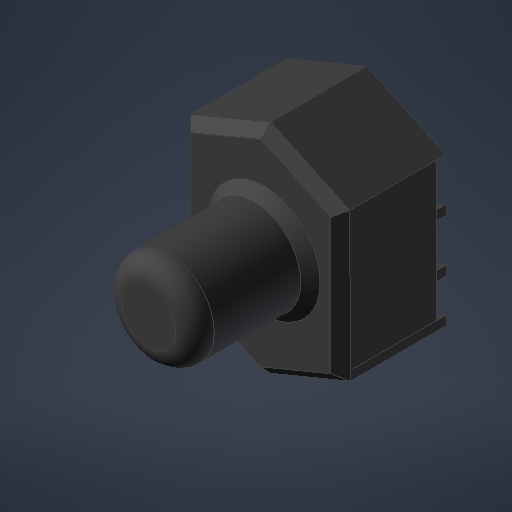
# Autodesk Inventor part: stamp
Saved by Autodesk Inventor 2026.1 (Build 301233000, 233)
## iProperties
Created: 2026-07-17
Part Number: stamp
Material: Generic
Document SubType Name: Modeling
Designer: aaron
Density: 1 g/cm^3
Appearance: Default
Author: aaron
Autodesk Inventor part; units mm, degrees
ref_plane "YZ Plane" through (0, 0, 0) normal (1, 0, 0) x (0, 1, 0)
ref_plane "XZ Plane" through (0, 0, 0) normal (0, 1, 0) x (-1, 0, 0)
ref_plane "XY Plane" through (0, 0, 0) normal (0, 0, 1) x (1, 0, 0)
sketch "Sketch1" plane through (0, 0, 0) normal (0, 0, 1) x (1, 0, 0)
  line L0 (7.712, 5.2132) -> (7.712, 6.1786)
  line L1 (7.712, 5.2132) -> (-0.617, 1.7442)
  line L2 (7.712, 6.1786) -> (-0.617, 2.7096)
  line L3 (-0.617, 7.1917) -> (7.712, 10.6607)
  line L4 (7.712, 10.6607) -> (-0.5182, 14.502)
  line L5 (-8.8472, 2.0687) -> (-8.8472, 6.5508)
  line L6 (-8.8472, 11.033) -> (-0.617, 7.1917)
  line L7 (-0.5182, 14.502) -> (-8.8472, 11.033)
  line L8 (-0.617, 2.7096) -> (-8.8472, 6.5508)
  line L9 (7.748, -0.2344) -> (7.748, 0.731)
  line L10 (-0.617, 1.7442) -> (-0.617, -1.7726)
  line L11 (7.748, 0.731) -> (-0.5892, -2.738)
  line L12 (7.748, -0.2344) -> (-0.617, -3.7034)
  line L13 (-0.617, -1.7726) -> (-8.8472, 2.0687)
  line L14 (-0.5892, -2.738) -> (-8.8472, 1.1033)
  line L15 (-8.8472, -4.2851) -> (-8.8472, 1.1033)
  line L16 (7.748, -4.7166) -> (7.748, -3.7512)
  line L17 (7.748, -3.7512) -> (-0.617, -7.2201)
  line L18 (-0.617, -8.1855) -> (7.748, -4.7166)
  line L19 (-0.617, -3.7034) -> (-0.617, -7.2201)
  line L20 (-0.617, -8.1855) -> (-8.8472, -4.2851)
  point P0 (0, 0)
  constraints: 42 end point, 1 point on line
extrude "Extrusion1" add sketch "Sketch1" along normal blind 1
sketch "Sketch2" plane through (0, 0, 1) normal (0, 0, 1) x (1, 0, 0)
  line L0 (-0.617, 7.1917) -> (7.712, 10.6607) projected
  line L1 (7.712, 10.6607) -> (-0.5182, 14.502) projected
  line L2 (-0.5182, 14.502) -> (-8.8472, 11.033) projected
  line L3 (-8.8472, 11.033) -> (-0.617, 7.1917) projected
  line L4 (7.748, -0.2344) -> (7.748, 0.731) projected
  line L5 (7.748, 0.731) -> (-0.5892, -2.738) projected
  line L6 (-0.5892, -2.738) -> (-8.8472, 1.1033) projected
  line L7 (-8.8472, 1.1033) -> (-8.8472, -4.2851) projected
  line L8 (-8.8472, -4.2851) -> (-0.617, -8.1855) projected
  line L9 (-0.617, -8.1855) -> (7.748, -4.7166) projected
  line L10 (7.748, -4.7166) -> (7.748, -3.7512) projected
  line L11 (7.748, -3.7512) -> (-0.617, -7.2201) projected
  line L12 (-0.617, -7.2201) -> (-0.617, -3.7034) projected
  line L13 (-0.617, -3.7034) -> (7.748, -0.2344) projected
  line L14 (-8.8472, 11.033) -> (-8.8472, 1.1033)
  line L15 (7.712, 10.6607) -> (7.748, -3.7512)
  point P0 (0, 0)
  constraints: 4 end point
extrude "Extrusion2" add sketch "Sketch2" along normal blind 10 contours L3 L2 L1 L0 | L0 L15 L5 L6 L14 L3 | L15 L13 L12 L11 L10 L9 L8 L7 L6 L5 | L15 L11 L12 L13
sketch "Sketch3" plane through (0, 0, 11) normal (0, 0, 1) x (1, 0, 0)
  circle A0 centre (-0.2029, 3.5969) radius 4.8142
  point P0 (0, 0)
  constraints: 1 centre point
extrude "Extrusion3" add sketch "Sketch3" along normal blind 12
fillet "Fillet1" radius 2 1 edges at (-5.0171, 3.5969, 23)
chamfer "Chamfer1" distance 1 angle 45 7 edges at (-8.8472, 3.374, 11) (-4.7321, -6.2353, 11) (3.5655, -6.451, 11) (7.73, 3.4548, 11) (3.5969, 12.5813, 11) (-4.6827, 12.7675, 11) (-5.0171, 3.5969, 11)
body "Solid1"
